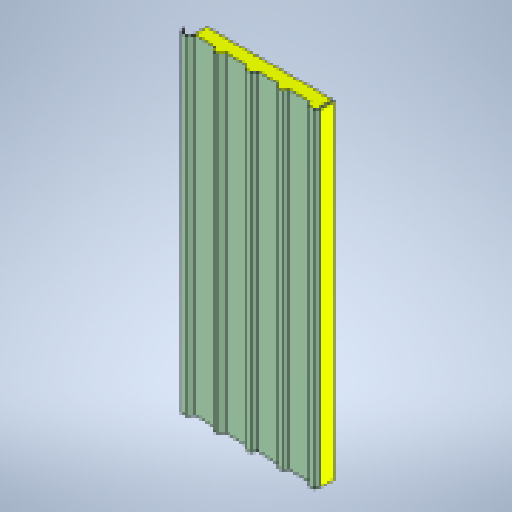
# Autodesk Inventor part: Sandwich 5  roof long
Saved by Autodesk Inventor 2025 (Build 290162010, 162A)
## iProperties
Created: 2022-10-17
Part Number: Sandwich 5  roof long
Material: Generic
Document SubType Name: Modeling
Designer: user
Density: 1 g/cm^3
Appearance: Rubber - Green
Author: user
Autodesk Inventor part; units mm, degrees
ref_plane "YZ Plane" through (0, 0, 0) normal (1, 0, 0) x (0, 1, 0)
ref_plane "XZ Plane" through (0, 0, 0) normal (0, 1, 0) x (-1, 0, 0)
ref_plane "XY Plane" through (0, 0, 0) normal (0, 0, 1) x (1, 0, 0)
sketch "Sketch1" plane through (0, 0, 0) normal (0, 0, 1) x (1, 0, 0)
  line L0 (-500, 1300) -> (500, 1300)
  line L1 (500, 1300) -> (500, -1300)
  line L2 (500, -1300) -> (-500, -1300)
  line L3 (-500, -1300) -> (-500, 1300)
  line L4 (-500, 1300) -> (500, -1300) construction
  line L5 (500, 1300) -> (-500, -1300) construction
  point P0 (0, 0)
  dimension "d0" = 1000
  dimension "d1" = 2600
  constraints: 12 end point, 2 midpoint, 2 parallel, 1 horizontal, 1 perpendicular
  measures "d0" distance of L1.end L2.end
  measures "d1" distance of L0.end L1.end
extrude "Extrusion1" add sketch "Sketch1" along normal blind 100
sketch "Sketch2" plane through (-500, -1300, 0) normal (0, -1, 0) x (1, 0, 0)
  line L0 (0, 0) -> (1000, 0) projected
  line L1 (1000, 0) -> (1000, 100) projected
  line L2 (0, 100) -> (1000, 100) projected
  line L3 (0, 0) -> (0, 100) projected
  line L4 (0, 100) -> (1000, 100) projected
  line L5 (1000, 100) -> (977, 135)
  line L6 (977, 135) -> (937, 135)
  line L7 (937, 135) -> (914, 100)
  line L8 (687, 135) -> (664, 100)
  line L9 (727, 135) -> (687, 135)
  line L10 (750, 100) -> (727, 135)
  line L11 (437, 135) -> (414, 100)
  line L12 (477, 135) -> (437, 135)
  line L13 (500, 100) -> (477, 135)
  line L14 (187, 135) -> (164, 100)
  line L15 (227, 135) -> (187, 135)
  line L16 (250, 100) -> (227, 135)
  line L17 (-63, 135) -> (-86, 100)
  line L18 (-23, 135) -> (-63, 135)
  line L19 (0, 100) -> (-23, 135)
  line L20 (-90.1785, 102.7459) -> (-65.6973, 140)
  line L21 (-65.6973, 140) -> (-20.3027, 140)
  line L22 (-20.3027, 140) -> (5.983, 100)
  line L23 (-90.1785, 102.7459) -> (-86, 100)
  point P0 (500, 0)
  point P1 (5.983, 100)
  dimension "d4" = 86
  dimension "d5" = 40
  dimension "d6" = 35
  dimension "d11" = 250
  dimension "d16" = 5
  dimension "d17" = 5
  constraints: 38 end point, 2 parallel, 2 point on line, 1 equal length, 1 horizontal, 29 other
  measures "d4" distance of L1.end L7.end
  measures "d5" distance of L5.end L6.end
  measures "d6" distance between parallel lines of L2 L6
  measures "d11" distance of L6.end L8.start
  measures "d16" distance between parallel lines of L17 L20
  measures "d17" distance between parallel lines of L19 L22
extrude "Extrusion2" add sketch "Sketch2" against normal up to surface (2600 mm away) contours L19 L18 L17 L23 L20 L21 L22 L2 | L2 L7 L6 L5 | L14 L15 L16 L2 | L2 L8 L9 L10 | L11 L12 L13 L2
chamfer "Chamfer1" distance 10 angle 45 2 edges at (500, -1300, 50) (500, 1300, 50)
equation "\"d17\" = d16"
body "Solid1"
